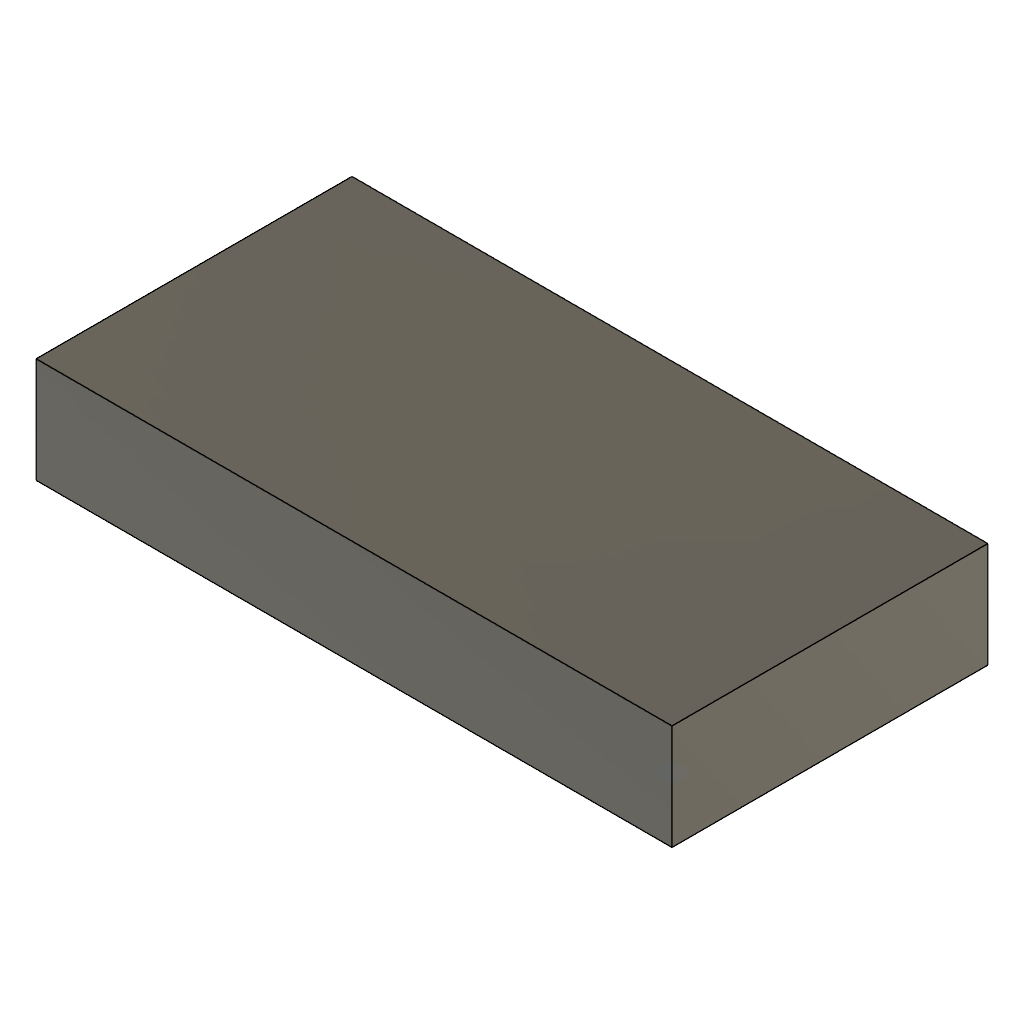
MacroPad (Autodesk Fusion 360 design; units mm, degrees)
part number: 2026-09-07-22-00-43-772
Autodesk Fusion 360 part; units mm, degrees
sketch "Sketch3" plane through (0, 0, 0) normal (0, 0, 1) x (1, 0, 0)
  line L0 (0, 0) -> (58.5, 0)
  line L1 (58.5, 0) -> (58.5, 19)
  line L2 (58.5, 19) -> (0, 19)
  line L3 (0, 19) -> (0, 0)
  dimension "d1" = 58.5
  dimension "d2" = 19
  constraint horizontal L0
  constraint vertical L1
  constraint horizontal L2
  constraint vertical L3
  constraint coincident L0.start L3.end
  measures "d1" distance of L0.start L0.end
  measures "d2" distance of L0.start L2.end
sketch "Sketch6" plane through (0, 0, 0) normal (0, 0, 1) x (1, 0, 0)
  line L0 (-10, -10) -> (68.5, -10)
  line L1 (68.5, -10) -> (68.5, 29)
  line L2 (68.5, 29) -> (-10, 29)
  line L3 (-10, 29) -> (-10, -10)
  dimension "d5" = 78.5
  dimension "d6" = 39
  constraint horizontal L0
  constraint vertical L1
  constraint horizontal L2
  constraint vertical L3
  measures "d5" distance of L0.start L0.end
  measures "d6" distance of L0.start L2.end
sketch "Sketch8" plane through (0, 0, 0) normal (0, 0, 1) x (1, 0, 0)
  circle A0 centre (-5, 24) radius 1.45
  circle A1 centre (-5, -5) radius 1.45
  circle A2 centre (63.5, -5) radius 1.45
  circle A3 centre (63.5, 24) radius 1.45
  dimension "d7" = 2.9
  dimension "d8" = 2.9
  dimension "d9" = 2.9
  dimension "d10" = 2.9
  measures "d7" diameter of A0
  measures "d8" diameter of A1
  measures "d9" diameter of A2
  measures "d10" diameter of A3
extrude "Extrude1" add sketch "Sketch6" along normal blind 13 makes body 1
extrude "Extrude2" cut sketch "Sketch3" along normal blind 10 bodies 1
extrude "Extrude3" cut sketch "Sketch8" along normal blind 3 bodies 1
sketch "plate-2026-09-07T15_19_25.806Z" plane through (0, 0, 0) normal (0, 0, 1) x (1, 0, 0)
  line L0 (3.025, 16.475) -> (16.025, 16.475)
  line L1 (3.025, 2.475) -> (16.025, 2.475)
  line L2 (2.525, 15.975) -> (2.525, 2.975)
  line L3 (16.525, 15.975) -> (16.525, 2.975)
  arc A0 (3.025, 16.475) -> (2.525, 15.975) centre (3.025, 15.975) ccw
  arc A1 (16.525, 15.975) -> (16.025, 16.475) centre (16.025, 15.975) ccw
  arc A2 (2.525, 2.975) -> (3.025, 2.475) centre (3.025, 2.975) ccw
  arc A3 (16.025, 2.475) -> (16.525, 2.975) centre (16.025, 2.975) ccw
  line L4 (22.075, 16.475) -> (35.075, 16.475)
  line L5 (22.075, 2.475) -> (35.075, 2.475)
  line L6 (21.575, 15.975) -> (21.575, 2.975)
  line L7 (35.575, 15.975) -> (35.575, 2.975)
  arc A4 (22.075, 16.475) -> (21.575, 15.975) centre (22.075, 15.975) ccw
  arc A5 (35.575, 15.975) -> (35.075, 16.475) centre (35.075, 15.975) ccw
  arc A6 (21.575, 2.975) -> (22.075, 2.475) centre (22.075, 2.975) ccw
  arc A7 (35.075, 2.475) -> (35.575, 2.975) centre (35.075, 2.975) ccw
  line L8 (41.125, 16.475) -> (54.125, 16.475)
  line L9 (41.125, 2.475) -> (54.125, 2.475)
  line L10 (40.625, 15.975) -> (40.625, 2.975)
  line L11 (54.625, 15.975) -> (54.625, 2.975)
  arc A8 (41.125, 16.475) -> (40.625, 15.975) centre (41.125, 15.975) ccw
  arc A9 (54.625, 15.975) -> (54.125, 16.475) centre (54.125, 15.975) ccw
  arc A10 (40.625, 2.975) -> (41.125, 2.475) centre (41.125, 2.975) ccw
  arc A11 (54.125, 2.475) -> (54.625, 2.975) centre (54.125, 2.975) ccw
  line L12 (0, -0.05) -> (57.15, -0.05)
  line L13 (0, 19) -> (57.15, 19)
  line L14 (0, -0.05) -> (0, 19)
  line L15 (57.15, 19) -> (60, 19)
  line L16 (60, 19) -> (60, 0)
  line L17 (60, 0) -> (57.15, -0.05)
  constraint parallel L13 L15
  constraint perpendicular L15 L16
extrude "Extrude4" add sketch "plate-2026-09-07T15_19_25.806Z" along normal blind 3 separate body makes body 2
sketch "Sketch10" plane through (0, 0, 3) normal (0, 0, -1) x (1, 0, 0)
  circle A0 centre (63.5, 5) radius 1.45
sketch "Sketch1" plane through (0, 0, 0) normal (0, 0, 1) x (1, 0, 0)
sketch "Sketch2" plane through (0, 0, 0) normal (0, 0, 1) x (1, 0, 0)
